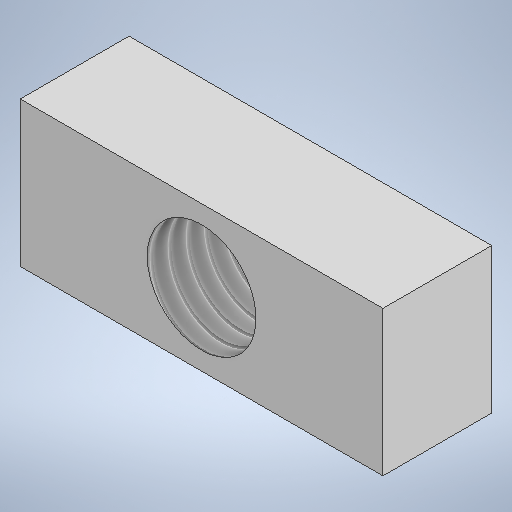
# Autodesk Inventor part: 19
Saved by Autodesk Inventor 2025.1 (Build 291241000, 241)
## iProperties
Created: 2024-09-13
Part Number: 19
Material: Generisch
Document SubType Name: Modeling
Designer: ffogue
Density: 1 g/cm^3
Appearance: Vorgabe
Author: ffogue
Autodesk Inventor part; units mm, degrees
ref_plane "YZ Plane" through (0, 0, 0) normal (1, 0, 0) x (0, 1, 0)
ref_plane "XZ Plane" through (0, 0, 0) normal (0, 1, 0) x (-1, 0, 0)
ref_plane "XY Plane" through (0, 0, 0) normal (0, 0, 1) x (1, 0, 0)
sketch "Sketch1" plane through (0, 0, 0) normal (0, 0, 1) x (1, 0, 0)
  line L0 (-5, -1.5) -> (5, -1.5)
  line L1 (5, -1.5) -> (5, 1.5)
  line L2 (5, 1.5) -> (-5, 1.5)
  line L3 (-5, 1.5) -> (-5, -1.5)
  line L4 (-5, -1.5) -> (5, 1.5) construction
  line L5 (5, -1.5) -> (-5, 1.5) construction
  point P0 (0, 0)
  dimension "d0" = 3
  dimension "d1" = 10
  constraints: 12 end point, 2 midpoint, 2 parallel, 1 horizontal, 1 perpendicular
  measures "d0" distance of L2.end L0.start
  measures "d1" distance of L1.end L2.end
extrude "Extrusion1" add sketch "Sketch1" along normal blind 4
sketch "Sketch2" plane through (-5, 1.5, 0) normal (0, 1, 0) x (1, 0, 0)
  circle A0 centre (5, -2) radius 1.5
  line L0 (0, 0) -> (0, -4) projected
  line L1 (10, 0) -> (0, 0) projected
  point P0 (5, 0)
  point P1 (0, -2)
  point P2 (5, 0)
  dimension "d4" = 3
  constraints: 2 midpoint, 1 centre point, 1 horizontal alignment, 1 vertical alignment
  measures "d4" diameter of A0
extrude "Extrusion2" cut sketch "Sketch2" against normal up to surface (3 mm away)
thread "Thread1" size "M3x0.5" class "6H" standard "ISO Metric profile" length 35.9
body "Solid1"
